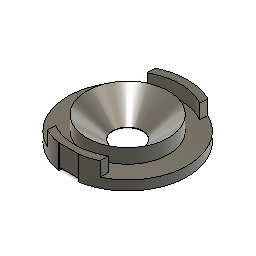
Bottom_Casing (Autodesk Fusion 360 design; units mm, degrees)
Autodesk Fusion 360 part; units mm, degrees
sketch "Sketch1" plane through (0, 0, 0) normal (0, 1, 0) x (1, 0, 0)
  circle A0 centre (0, 0) radius 25
  dimension "d6" = 50
  measures "d6" diameter of A0
extrude "Extrude1" add sketch "Sketch1" along normal blind 10
sketch "Sketch4" plane through (0, 10, 0) normal (0, 1, 0) x (-1, 0, 0)
  circle A0 centre (0, 0) radius 25
  circle A1 centre (0, 0) radius 21
  dimension "d10" = 42
  constraint coincident A0.centre A1.centre
  measures "d10" diameter of A1
extrude "Extrude2" cut sketch "Sketch4" against normal blind 8 contours A1
sketch "Sketch5" plane through (0, 2, 0) normal (0, 1, 0) x (-1, 0, 0)
  circle A0 centre (0, 0) radius 21
  circle A1 centre (0, 0) radius 17
  dimension "d13" = 34
  constraint concentric A0 A1
  measures "d13" diameter of A1
extrude "Extrude3" add sketch "Sketch5" along normal blind 8 contours A1
sketch "Sketch6" plane through (0, 10, 0) normal (0, 1, 0) x (-1, 0, 0)
  circle A0 centre (0, 0) radius 17
  circle A1 centre (0, 0) radius 15
  dimension "d16" = -2
extrude "Extrude4" cut sketch "Sketch6" against normal blind 8 contours A1
sketch "Sketch7" plane through (0, 2, 0) normal (0, 1, 0) x (-1, 0, 0)
  circle A0 centre (0, 0) radius 15
extrude "Extrude8" add 1 faces at (-0.9463, 2, -5.6032) along direction (0, 1, 0) blind 5
sketch "Sketch12" plane through (0, 7, 0) normal (0, 1, 0) x (-1, 0, 0)
  circle A0 centre (0, 0) radius 15
ref_plane "WorkPlane1" through (0, 0, 0) normal (0, -1, 0) x (-1, 0, 0)
sketch "Sketch13" plane through (0, 0, 0) normal (0, -1, 0) x (1, 0, 0)
  circle A0 centre (0, 0) radius 5
  dimension "d36" = 10
  constraint coincident A0.centre origin
  measures "d36" diameter of A0
extrude "Extrude9" add sketch "Sketch12" along normal blind 3
loft "Loft1" cut profiles "Sketch13" section 1 face at (-5.4149, 10, 3.2471) section 2
sketch "Sketch14" plane through (0, 0, 0) normal (0, -1, 0) x (1, 0, 0)
  circle A0 centre (0, 0) radius 5
  circle A1 centre (0, 0) radius 25
  circle A2 centre (0, 0) radius 6.5
  dimension "d39" = 1.5
extrude "Extrude10" cut sketch "Sketch14" against normal blind 1 contours A2
extrude "Extrude11" add 1 faces at (-19.5252, 2, -1.8879) along direction (0, 1, 0) blind 7
extrude "Extrude12" cut 1 faces at (-19.5252, 9, -1.8879) along direction (0, -1, 0) blind 5
sketch "Sketch15" plane through (0, 10, 0) normal (0, 1, 0) x (-1, 0, 0)
  circle A0 centre (0, 0) radius 21
  circle A1 centre (0, 0) radius 25
  line L0 (-11.0532, -17.8557) -> (-11.0532, -22.4238)
  line L1 (10.9663, -17.9092) -> (10.9663, -22.4664)
  arc A2 (-11.0532, -17.8557) -> (10.9663, -17.9092) centre (0, 0) ccw
  arc A3 (-11.0532, -22.4238) -> (10.9663, -22.4664) centre (0, 0) ccw
  arc A4 (11.0532, 22.4238) -> (-10.9663, 22.4664) centre (0, 0) ccw
  line L2 (11.0532, 17.8557) -> (11.0532, 22.4238)
  arc A5 (11.0532, 17.8557) -> (-10.9663, 17.9092) centre (0, 0) ccw
  line L3 (-10.9663, 17.9092) -> (-10.9663, 22.4664)
  dimension "d47" = 360
  constraint vertical L0
  constraint coincident A0 L0.start
  constraint coincident A1 L0.end
  constraint coincident A0 L1.start
  constraint coincident A1 L1.end
  constraint vertical L1
extrude "Extrude13" cut sketch "Sketch15" against normal blind 6 contours A0 A1 L1 L2 | A0 A1 L0 L3
move_face "OffsetFaces1" offset -1 1 faces at (6.6925, 6, -19.905)
move_face "OffsetFaces2" offset -1 1 faces at (6.5958, 8, 19.9373)
sketch "Sketch20" plane through (0, 0, 0) normal (0, -1, 0) x (1, 0, 0)
  circle A0 centre (0, 0) radius 6.5
  circle A1 centre (0, 0) radius 25
  circle A2 centre (0, 0) radius 7.5
  dimension "d70" = 1
extrude "Extrude18" cut sketch "Sketch20" against normal blind 1 contours A2
sketch "Sketch23" plane through (0, 0, 0) normal (0, -1, 0) x (1, 0, 0)
  line L0 (2.5124, 8.3759) -> (-2.4876, 8.3759)
  line L1 (-2.4876, 8.3759) -> (-2.4876, 13.3759)
  line L2 (-2.4876, 13.3759) -> (2.5124, 13.3759)
  line L3 (2.5124, 13.3759) -> (2.5124, 8.3759)
  line L4 (2.5124, 8.3759) -> (-2.4876, 13.3759) construction
  line L5 (-2.4876, 8.3759) -> (2.5124, 13.3759) construction
  circle A0 centre (0, 0) radius 25
  circle A1 centre (0, 0) radius 7.5
  circle A2 centre (0, 0) radius 25
  point P0 (0.0124, 10.8759)
  dimension "d77" = 5
  dimension "d78" = 5
  constraint horizontal L0
  constraint perpendicular L0 L1
  constraint parallel L0 L2
  constraint parallel L1 L3
  constraint coincident L4 P0
  constraint coincident L5 P0
  measures "d77" distance of L1.end L2.end
  measures "d78" distance of L0.end L1.end
extrude "Extrude19" cut sketch "Sketch23" against normal blind 1 contours L0 L1 L2 L3
extrude "Extrude23" add 2 faces at (7.1387, 1, -0.3726) (6.3527, 1, -0.6309) along direction (0, -1, 0) blind 0.2
ref_plane "WorkPlane5" through (0, 4.8995, 25) normal (0, 0, 1) x (-1, 0, 0)
sketch "Sketch26" plane through (0, 4.8995, 25) normal (0, 0, 1) x (1, 0, 0)
  arc A0 through (-5.6622, 5.1005, -0.6497) (0, 5.1005, 0) (5.6622, 5.1005, -0.6497)
  arc A1 through (10.9663, 5.1005, -2.5336) (-0.0484, 5.1005, 0) (-11.0532, 5.1005, -2.5762)
  circle A2 through (25, -4.8995, -25) (-12.5, -4.8995, -3.3494) (-12.5, -4.8995, -46.6506)
  line L0 (-5.6622, 5.1005, -0.6497) -> (-5.6622, -4.8995, -0.6497)
  line L1 (5.6622, 5.1005, -0.6497) -> (5.6622, -4.8995, -0.6497)
  arc A3 through (5.6622, -4.8995, -0.6497) (0, -4.8995, 0) (-5.6622, -4.8995, -0.6497)
  line L2 (4, -5) -> (-4, -5)
  line L3 (-4, -5) -> (-4, 5)
  line L4 (-4, 5) -> (4, 5)
  line L5 (4, 5) -> (4, -5)
  line L6 (4, -5) -> (-4, 5) construction
  line L7 (-4, -5) -> (4, 5) construction
  constraint horizontal L2
  constraint perpendicular L2 L3
  constraint parallel L2 L4
  constraint parallel L3 L5
  constraint coincident L6 origin
  constraint coincident L7 origin
extrude "Extrude25" cut sketch "Sketch26" against normal blind 1
extrude "Extrude26" cut 1 faces at (-0.4461, 9.8995, 24.3214) along direction (0, 1, 0) through all
sketch "Sketch27" plane through (0, 0, 0) normal (0, -1, 0) x (1, 0, 0)
  line L0 (-4, 24) -> (-4, 24.6779)
  arc A0 (-4, 24.6779) -> (4, 24.6779) centre (0, 0) ccw
  line L1 (4, 24.6779) -> (4, 24)
  line L2 (4, 24) -> (-4, 24)
  line L3 (-2.4876, 8.3759) -> (-2.4876, 13.3759)
  line L4 (-2.4876, 13.3759) -> (2.5124, 13.3759)
  line L5 (2.5124, 13.3759) -> (2.5124, 8.3759)
  line L6 (2.5124, 8.3759) -> (-2.4876, 8.3759)
  circle A1 centre (0, 0) radius 7.5
  line L7 (-4, 24) -> (4, 24)
  line L8 (4, 24) -> (4, 9.5)
  line L9 (4, 9.5) -> (-4, 9.5)
  line L10 (-4, 9.5) -> (-4, 24)
  constraint horizontal L7
  constraint vertical L8
  constraint horizontal L9
  constraint vertical L10
  constraint coincident L0.start L2.end
extrude "Extrude27" cut sketch "Sketch27" against normal blind 1 contours L2 L3 L4 L5 L7 L8 L9 L10
extrude "Extrude28" add 1 faces at (0.8457, 0.3333, 8.3759) along direction (0, 0, 1) blind 1.12
extrude "Extrude29" add 1 faces at (-0.8292, 1, 19.1667) along direction (0, -1, 0) blind 0.8
extrude "Extrude30" add 1 faces at (1.3333, 6.7333, 24) along direction (0, 0, 1) blind 0.5
fillet "Fillet1" radius 1 1 edges at (0, 0.2, 24.5)
component "Bottom Casing" placed x (1, 0, 0) y (0, 1, 0) z (0, 0, 1) at (0, 0, 0)
